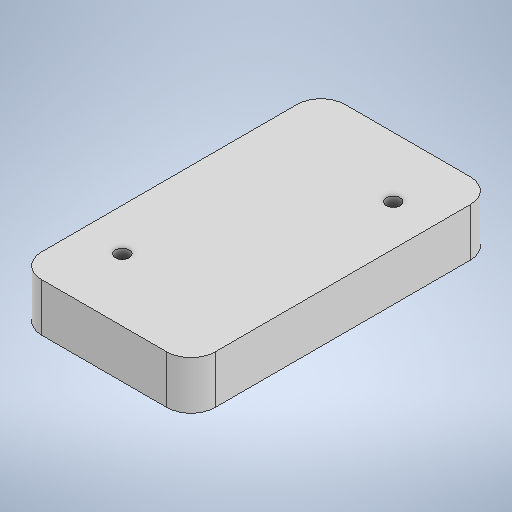
# Autodesk Inventor part: BASE BUCKBOOST
Saved by Autodesk Inventor 2025 (Build 290162000, 162)
## iProperties
Created: 2024-09-30
Part Number: BASE BUCKBOOST
Material: Genérico
Document SubType Name: Modeling
Designer: phmca
Density: 1 g/cm^3
Appearance: Padrão
Author: phmca
Autodesk Inventor part; units mm, degrees
ref_plane "YZ Plane" through (0, 0, 0) normal (1, 0, 0) x (0, 1, 0)
ref_plane "XZ Plane" through (0, 0, 0) normal (0, 1, 0) x (-1, 0, 0)
ref_plane "XY Plane" through (0, 0, 0) normal (0, 0, 1) x (1, 0, 0)
sketch "Esboço1" plane through (0, 0, 0) normal (0, 1, 0) x (-1, 0, 0)
  line L0 (13, 26.5) -> (-13, 26.5) construction
  line L1 (-13, 26.5) -> (-13, -26.5) construction
  line L2 (-13, -26.5) -> (13, -26.5) construction
  line L3 (13, -26.5) -> (13, 26.5) construction
  line L4 (-18, 31.5) -> (18, 31.5)
  line L5 (18, 31.5) -> (18, -31.5)
  line L6 (18, -31.5) -> (-18, -31.5)
  line L7 (-18, -31.5) -> (-18, 31.5)
  line L8 (-18, 31.5) -> (18, -31.5) construction
  line L9 (18, 31.5) -> (-18, -31.5) construction
  circle A0 centre (9.25, 18.5) radius 1.45
  circle A1 centre (-9.5, -19) radius 1.45
  point P0 (0, 0)
  dimension "d0" = 53
  dimension "d1" = 26
  dimension "d2" = 26.5
  dimension "d3" = 13
  dimension "d4" = 5
  dimension "d5" = 5
  dimension "d6" = 2.9
  dimension "d7" = 2.9
  dimension "d10" = 45
  dimension "d11" = 3.75
  dimension "d12" = 45.5
  dimension "d13" = 3.5
  constraints: 20 end point, 4 parallel, 2 centre point, 2 horizontal, 2 midpoint, 2 perpendicular
  measures "d0" distance of L2.end L0.start
  measures "d1" distance of L1.end L2.end
  measures "d2" distance from line of L2 point (0, 0)
  measures "d3" distance from line of L3 point (0, 0)
  measures "d4" distance between parallel lines of L5 L3
  measures "d5" distance between parallel lines of L0 L4
  measures "d6" diameter of A1
  measures "d7" diameter of A0
  measures "d10" distance from line of L2 A0.centre
  measures "d11" distance from line of L3 A0.centre
  measures "d12" distance from line of L0 A1.centre
  measures "d13" distance from line of L1 A1.centre
extrude "Extrusão1" add sketch "Esboço1" along normal blind 10 contours L4 L5 L6 L7 | A0 | A1
sketch "Esboço2" plane through (0, 10, 0) normal (0, 1, 0) x (1, 0, 0)
  circle A0 centre (-9.25, -18.5) radius 1.45 projected
  circle A1 centre (9.5, 19) radius 1.45 projected
  point P0 (0, 0)
extrude "Extrusão2" cut sketch "Esboço2" against normal blind 8.5
fillet "Arredondamento1" radius 5 4 edges at (18, 5, 31.5) (18, 5, -31.5) (-18, 5, -31.5) (-18, 5, 31.5)
equation "\"d2\" = 0.5 * d0"
equation "\"d3\" = 0.5 * d1"
equation "\"d7\" = d6"
